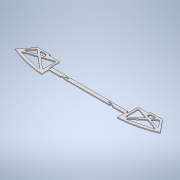
# Autodesk Inventor part: bulkhead_front_center
Saved by Autodesk Inventor 2022 (Build 260153000, 153)
## iProperties
Created: 2021-04-24
Part Number: bulkhead_front_center
Material: Generic
Document SubType Name: Modeling
Designer: kardo
Density: 1 g/cm^3
Appearance: Default
Mass: 7.4811 g
Surface Area: 102.002 cm^2
Volume: 7.4811 cm^3
Author: kardo
Autodesk Inventor part; units mm, degrees
ref_plane "YZ Plane" through (0, 0, 0) normal (1, 0, 0) x (0, 1, 0)
ref_plane "XZ Plane" through (0, 0, 0) normal (0, 1, 0) x (-1, 0, 0)
ref_plane "XY Plane" through (0, 0, 0) normal (0, 0, 1) x (1, 0, 0)
derived "frame_outline.ipt"
sketch "bh_front_center" plane through (0, 94.8, 0) normal (0, 1, 0) x (-1, 0, 0)
  line L0 (-156.125, 34.3232) -> (-133.5, 6.6291) construction
  line L1 (-133.5, 6.6291) -> (-81, 6.6291) construction
  line L2 (-81, 29.632) -> (0, 29.632)
  line L3 (-81, 36.736) -> (0, 36.736)
  line L4 (0, 36.736) -> (0, 29.632)
  line L5 (-81, 29.632) -> (-81, 7.4291)
  line L6 (-81, 6.6291) -> (-81, 6.6291) construction
  line L7 (-81, 7.4291) -> (-133.1205, 7.4291)
  line L8 (-133.1205, 7.4291) -> (-154.8407, 34.0156)
  line L9 (-81, 51.7967) -> (-81, 36.736)
  line L10 (-81, 7.4291) -> (-81, 6.6291) construction
  line L11 (-81, 29.632) -> (-81, 6.6291) construction
  spline S0 degree 3 poles (-81, 52.5981) (-93.8155, 51.8415) (-106.5454, 49.9821) (-131.8146, 43.8672) (-144.1829, 39.6271) (-156.125, 34.3232) knots 0 0 0 0 3.851348 3.851348 7.75462 7.75462 7.75462 7.75462
  spline S1 degree 3 poles (-154.8407, 34.0156) (-150.9488, 35.7222) (-144.0597, 38.5105) (-136.0383, 41.2888) (-130.4682, 43.0348) (-127.4113, 43.9308) (-124.3399, 44.7813) (-122.285, 45.3255) (-119.9656, 45.9118) (-118.4143, 46.2884) (-116.8616, 46.653) (-115.8255, 46.8901) (-114.2701, 47.2368) (-112.713, 47.5716) (-109.8544, 48.1581) (-106.7294, 48.7504) (-102.0303, 49.5502) (-97.8418, 50.167) (-92.5931, 50.8217) (-87.3322, 51.3612) (-83.1123, 51.6716) (-81, 51.7967) knots 0.00474 0.00474 0.00474 0.00474 1.278916 2.234547 2.553091 3.030907 3.190179 3.508723 3.667995 3.906903 3.986539 4.145811 4.225447 4.464354 4.623626 5.101442 5.419986 6.057074 6.375618 7.012706 7.649793 7.649793 7.649793 7.649793
  line L12 (-81, 10.5986) -> (-107.046, 10.5986)
  line L13 (-107.046, 10.5986) -> (-107.046, 7.4291)
  line L14 (-107.046, 5.1533) -> (-107.046, 0.8)
  point P0 (0, 0)
  point P1 (-81, 28.832)
  point P2 (-81, 37.536)
  point P3 (-81, 33.184)
ref_plane "plane_cowl" through (55, 0, 0) normal (1, 0, 0) x (0, 1, 0)
extrude "Extrusion1" add sketch "bh_front_center" against normal blind 2 contours L5 L12 L13 L7 L8 S1 L9 L3 L4 L2
sketch "Sketch4" plane through (0, 94.8, 29.632) normal (0, 1, 0) x (1, 0, 0)
  line L0 (55, 39.9913) -> (55, -32.5241) projected
  line L1 (81, -7.104) -> (0, -7.104) projected
  line L2 (55, -7.104) -> (55, -5.104)
  line L3 (55, -5.104) -> (49, -5.104)
  line L4 (49, -4.104) -> (49, -2.104)
  line L5 (49, -2.104) -> (43, -2.104)
  line L6 (43, -2.104) -> (43, -7.104)
  line L7 (49, -5.104) -> (49, -7.104)
  line L8 (0, -7.104) -> (81, -7.104) projected
  line L9 (49, -4.104) -> (43, -4.104)
  point P0 (0, 29.632)
  dimension "d15" = 2
  dimension "d16" = 5
  dimension "d17" = 6
  dimension "d18" = 6
  dimension "d21" = 2
  constraints: 14 end point, 6 point on line, 3 horizontal, 3 vertical, 1 collinear
  measures "d15" distance of L2.start L2.end
  measures "d16" distance of L5.end L6.end
  measures "d17" distance of L2.end L3.end
  measures "d18" distance of L4.end L5.end
  measures "d21" distance of L4.start L4.end
sketch "Sketch2" plane through (0, 94.8, 29.632) normal (0, 1, 0) x (1, 0, 0)
  line L0 (81, 19.0334) -> (81, 0) projected
  line L1 (133.1205, 22.2029) -> (107.046, 22.2029) projected
  line L2 (81, -3.552) -> (81, 0)
  line L3 (81, -3.552) -> (84, -3.552)
  line L4 (84, -3.552) -> (84, 22.2029)
  line L5 (84, 22.2029) -> (81, 22.2029)
  line L6 (81, 22.2029) -> (81, 19.0334)
  point P0 (0, 29.632)
  dimension "d3" = 3
  constraints: 10 end point, 2 horizontal, 1 collinear, 1 parallel, 1 point on line, 1 vertical
  measures "d3" distance between parallel lines of L0 L4
extrude "Extrusion2" cut sketch "Sketch2" against normal through all
sketch "Sketch3" plane through (0, 94.8, 36.736) normal (0, 1, 0) x (1, 0, 0)
  line L0 (154.8407, 2.7204) -> (133.1205, 29.3069) projected
  line L1 (84, 26.1374) -> (84, 3.552) projected
  line L2 (133.1205, 29.3069) -> (107.046, 29.3069) projected
  line L3 (133.1205, 29.3069) -> (154.8407, 2.7204) projected
  line L4 (154.8407, 2.7204) -> (84, 26.1374) construction
  line L5 (133.1205, 29.3069) -> (81, -15.0607) construction
  line L6 (146.2907, 3.4402) -> (89.553, -10.4065)
  line L7 (89.553, -10.4065) -> (117.1394, 13.0765)
  line L8 (117.1394, 13.0765) -> (146.2907, 3.4402)
  line L9 (145.4071, 7.9452) -> (120.7042, 16.111)
  line L10 (120.7042, 16.111) -> (131.3396, 25.1644)
  line L11 (131.3396, 25.1644) -> (145.4071, 7.9452)
  line L12 (121.6128, 22.1374) -> (116.2593, 17.5803)
  line L13 (116.2593, 17.5803) -> (102.4731, 22.1374)
  line L14 (102.4731, 22.1374) -> (121.6128, 22.1374)
  line L15 (112.6945, 14.5458) -> (88, -6.4755)
  line L16 (88, -6.4755) -> (88, 22.7087)
  line L17 (88, 22.7087) -> (112.6945, 14.5458)
  line L18 (89.553, -10.4065) -> (90.5013, -14.2925) construction
  line L19 (146.2907, 3.4402) -> (147.2391, -0.4457) construction
  line L20 (107.046, 26.1374) -> (84, 26.1374) projected
  line L21 (121.6128, 22.1374) -> (125.3361, 25.3069)
  line L22 (125.3361, 25.3069) -> (111.046, 25.3069)
  line L23 (111.046, 25.3069) -> (111.046, 22.1374)
  line L24 (107.046, 29.3069) -> (107.046, 26.1374) projected
  point P0 (0, 36.736)
  dimension "d7" = 4
  dimension "d8" = 4
  dimension "d9" = 4
  dimension "d10" = 4
  dimension "d12" = 4
  dimension "d23" = 4
  dimension "d24" = 4
  dimension "d25" = 4
  constraints: 38 end point, 6 parallel, 5 collinear, 2 horizontal, 2 perpendicular, 1 point on line, 6 other
  measures "d7" distance of L6.end L18.end
  measures "d8" distance between parallel lines of L8 L9
  measures "d9" distance between parallel lines of L15 L7
  measures "d10" distance between parallel lines of L0 L11
  measures "d12" distance between parallel lines of L1 L16
  measures "d23" distance between parallel lines of L20 L14
  measures "d24" distance between parallel lines of L24 L23
extrude "Extrusion3" cut sketch "Sketch3" against normal through all
extrude "Extrusion4" cut sketch "Sketch4" against normal through all
fillet "Fillet1" radius 1.3333 13 edges at (88, 93.8, 14.0273) (117.1394, 93.8, 23.6595) (102.4731, 93.8, 14.5986) (120.7042, 93.8, 20.625) (88, 93.8, 43.2115) (89.553, 93.8, 47.1425) (116.2593, 93.8, 19.1557) (112.6945, 93.8, 22.1902) (146.2907, 93.8, 33.2958) (145.4071, 93.8, 28.7908) (131.3396, 93.8, 11.5716) (125.3361, 93.8, 11.4291) (111.046, 93.8, 11.4291)
mirror "Mirror1" about plane through (0, 0, 0) normal (1, 0, 0)
equation "\"d1\" = bulkhead_thickness"
equation "\"d15\" = cowl_liner_thickness"
equation "\"d16\" = cowl_liner_thickness + cowl_insulation_thickness"
equation "\"d17\" = cowl_liner_width"
equation "\"d18\" = cowl_insulation_width"
equation "\"d21\" = cowl_liner_thickness"
equation "\"d3\" = stringer_thickness"
equation "\"d7\" = inset"
equation "\"d8\" = inset"
equation "\"d9\" = inset"
equation "\"d10\" = inset"
equation "\"d12\" = inset"
equation "\"d23\" = inset"
equation "\"d24\" = inset"
equation "\"d25\" = inset"
equation "\"d22\" = 0.333333 * inset"
equation "\"bulkhead_thickness\" = 2"
equation "\"cowl_liner_thickness\" = 2"
equation "\"cowl_insulation_thickness\" = 3"
equation "\"cowl_liner_width\" = 6"
equation "\"cowl_insulation_width\" = 6"
equation "\"stringer_thickness\" = 3"
equation "\"inset\" = 4"
body "Solid1"
